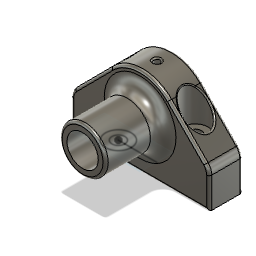
JKK60_WithCover_RailAdapter_12mm v9 (Autodesk Fusion 360 design; units mm, degrees)
Autodesk Fusion 360 part; units mm, degrees
note: some values were not read from the file. Chosen so that the rebuilt part matches the saved one: which face or edge a step refers to. Set by a fixed rule: which sketch regions a step uses.
sketch "Skizze1" plane through (0, 0, 0) normal (0, 0, 1) x (1, 0, 0)
  circle A0 centre (0, 0) radius 6
  line L0 (-27, -18.5) -> (0, -18.5)
  circle A1 centre (0, 0) radius 16
  line L1 (-27, -18.5) -> (-27, -4.5)
  line L2 (-27, -4.5) -> (-11.3594, 11.2678)
  line L3 (0, -18.5) -> (0, 0)
  circle A2 centre (0, 0) radius 16.5 construction
  line L4 (0, -16.5) -> (21.529, -16.5)
  line L5 (0, 0) -> (0, 20)
  circle A3 centre (62.865, -3.5125) radius 6
  circle A4 centre (62.865, -3.5125) radius 12.5
  line L6 (62.865, -3.5125) -> (62.865, -24.0125)
  line L7 (62.365, -24.0125) -> (92.365, -24.0125)
  circle A5 centre (62.865, -3.5125) radius 16.5 construction
  line L8 (62.865, -20.0125) -> (75, -20.0125) construction
  line L9 (50.365, -24.0125) -> (62.365, -24.0125)
  line L10 (92.365, -24.0125) -> (104.365, -24.0125)
  line L11 (68.6713, 7.5571) -> (104.365, -11.1649)
  line L12 (104.365, -11.1649) -> (104.365, -24.0125)
  line L13 (50.365, -3.5125) -> (50.365, -24.0125)
  point P0 (-15, -18.5)
  dimension "d1" = 12
  dimension "d3" = 32
  dimension "d4" = 33
  dimension "d5" = 2
  dimension "d6" = 27
  dimension "d7" = 15
  dimension "d8" = 12
  dimension "d9" = 25
  dimension "d10" = 30
  dimension "d11" = 33
  dimension "d12" = 4
  dimension "d13" = 54
  dimension "d14" = 12.8476
  dimension "d25" = 14
  constraint coincident A0.centre A1.centre
  constraint horizontal L0
  constraint concentric A0 A1
  constraint perpendicular L0 L1
  constraint vertical L3
  constraint concentric A0 A2
  constraint coincident L3 L4.start
  constraint perpendicular L3 L4
  constraint tangent A2 L4
  constraint coincident A1 L2.end
  constraint tangent A1 L2
  constraint coincident L0 P0
  constraint parallel L3 L5
  constraint concentric A3 A4
  constraint coincident A3.centre A4.centre
  constraint vertical L6
  constraint horizontal L7
  constraint coincident L6.end L7
  constraint concentric A4 A5
  constraint coincident L6 L8.start
  constraint perpendicular L6 L8
  constraint tangent A5 L8
  constraint perpendicular L6 L9
  constraint coincident L7.start L9.end
  constraint parallel L7 L10
  constraint equal L9 L10
  constraint coincident A4 L11.start
  constraint perpendicular L10 L12
  constraint tangent A4 L11
  constraint coincident A4 L13.start
  constraint vertical L13
  constraint tangent A4 L13
  measures "d1" diameter of A0
  measures "d3" diameter of A1
  measures "d4" diameter of A2
  measures "d5" distance of L0 L4
  measures "d6" distance of L0.start L0.end
  measures "d7" distance of L0.end P0
  measures "d8" diameter of A3
  measures "d9" diameter of A4
  measures "d10" distance of L7.start L7.end
  measures "d11" diameter of A5
  measures "d12" distance of L7 L8
  measures "d13" distance of L9.start L10.end
  measures "d14" distance of L10.end L11.end
  measures "d25" distance of L0.start L1.end
extrude "Extrusion1" add sketch "Skizze1" along normal blind 13 contours A0 A1 L3 L5 | L0 A1 L1 L2 L3 picked at (-9.646, 8.1637)
sketch "Skizze2" plane through (0, -18.5, 0) normal (0, -1, 0) x (1, 0, 0)
  line L0 (-27, 0) -> (0, 0)
  line L1 (0, 0) -> (0, 13)
  line L2 (0, 13) -> (-27, 13)
  line L3 (-27, 13) -> (-27, 0)
  line L4 (0, 6.5) -> (-15, 6.5)
  circle A0 centre (-15, 6.5) radius 2.5
  circle A1 centre (-15, 6.5) radius 5
  dimension "d17" = 5
  dimension "d18" = 10
  dimension "d37" = 15
  constraint midpoint L1 L4.start
  constraint perpendicular L1 L4
  constraint coincident L4.end A0.centre
  constraint concentric A0 A1
  measures "d17" diameter of A0
  measures "d18" diameter of A1
  measures "d37" distance of L4.start L4.end
extrude "Extrusion2" cut sketch "Skizze2" against normal blind 27 contours A0
ref_plane "Arbeitsebene1" through (-13.5, -1.5, 6.5) normal (0, -1, 0) x (1, 0, 0)
extrude "Extrusion3" cut sketch "Skizze2" against normal blind 27 from surface at -17 contours A0 | A1
mirror "Spiegeln1" about plane through (0, -16, 0) normal (1, 0, 0) of bodies 1 merged
sketch "Skizze3" plane through (11.3594, 11.2678, 0) normal (0.709965, 0.704237, 0) x (0, 0, -1)
  line L0 (0, -22.2092) -> (0, 0)
  line L1 (-9.9273, 0) -> (-13, 0)
  line L2 (-13, 0) -> (-13, -22.2092)
  line L3 (-13, -22.2092) -> (0, -22.2092)
  line L4 (0, -6) -> (0, 6)
  line L5 (0, 0) -> (-6.5, 0)
  circle A0 centre (-6.5, 0) radius 1.25
  line L6 (-6.5, 0) -> (-6.5, 5.407)
  ellipse E0 centre (-6.5, -5.1695) end of major axis (-6.5, 1.9304) minor radius 5 (-9.9273, 0) -> (-3.0727, 0) ccw
  line L7 (0, 0) -> (-3.0727, 0)
  dimension "d28" = 2.5
  constraint coincident L4 L0.end
  constraint perpendicular L4 L5
  constraint symmetric L4.start L4.end L5
  constraint coincident L5.end A0.centre
  constraint perpendicular L1 L6
  constraint symmetric L1.end L0.end L6
  measures "d28" diameter of A0
sketch "Skizze5" plane through (0, 0, 13) normal (0, 0, 1) x (1, 0, 0)
  arc A0 (11.3594, 11.2678) -> (-11.3594, 11.2678) centre (0, 0) ccw
  line L0 (-11.3594, 11.2678) -> (-27, -4.5)
  line L1 (-27, -4.5) -> (-27, -18.5)
  line L2 (-27, -18.5) -> (27, -18.5)
  line L3 (27, -18.5) -> (27, -4.5)
  line L4 (27, -4.5) -> (11.3594, 11.2678)
  circle A1 centre (0, 0) radius 6
  circle A2 centre (0, 0) radius 9
  dimension "d46" = 18
  constraint coincident A0.centre A1.centre
  measures "d46" diameter of A2
ref_plane "Arbeitsebene3" through (0, -1.25, 6.5) normal (0, 0, -1) x (-1, 0, 0)
ref_plane "Arbeitsebene4" through (0, -1.25, 35.5) normal (0, 0, -1) x (-1, 0, 0)
extrude "Extrusion6" add sketch "Skizze5" along normal up to surface (22.5 mm away) contours A2
fillet "Abrundung1" radius 5 2 edges at (-27, -4.5, 6.5) (27, -4.5, 6.5)
fillet "Abrundung6" radius 5 1 edges at (-8.3909, 3.2545, 13)
sketch "Skizze6" plane through (0, 0, 35.5) normal (0, 0, 1) x (1, 0, 0)
  circle A0 centre (0, 0) radius 6
  circle A1 centre (0, 0) radius 9
  circle A2 centre (0, 0) radius 6.1
  dimension "d52" = 0.1
extrude "Extrusion7" cut sketch "Skizze6" against normal up to surface (22.5 mm away) contours A0 | A2
fillet "Abrundung2" radius 1 19 edges at (27, -12.5296, 13) (0, -18.5, 13) (-27, -12.5296, 13) (-26.6233, -4.6552, 13) (-18.4546, 4.1149, 13) (0, 16, 13) (18.4546, 4.1149, 13) (26.6233, -4.6552, 13) (27, -12.5296, 0) (0, -18.5, 0) (-27, -12.5296, 0) (-26.6233, -4.6552, 0) (-18.4546, 4.1149, 0) (0, 16, 0) (18.4546, 4.1149, 0) (26.6233, -4.6552, 0) (-9, 0, 35.5) (6, 0, 0) (-6, 0, 0)
fillet "Abrundung5" radius 0.5 4 edges at (-10, 12.49, 6.5) (-20, 2.5569, 6.5) (10, 12.49, 6.5) (20, 2.5569, 6.5)
ref_plane "Arbeitsebene2" through (0, 21.5, 6.5) normal (0, -1, 0) x (1, 0, 0)
sketch "Skizze4" plane through (0, 21.5, 0) normal (0, -1, 0) x (-1, 0, 0)
  circle A0 centre (0, -6.5) radius 1.25
  point P0 (0, -6.5)
  dimension "d39" = 2.5
  constraint coincident P0 A0.centre
  measures "d39" diameter of A0
extrude "Extrusion5" cut sketch "Skizze4" along normal blind 19
fillet "Abrundung4" radius 0.5 1 edges at (-1.25, 15.9511, 6.5)
equation "d3 = d1 + 20 mm"
equation "d6 = ( 54 / 2 ) * 1 mm"
equation "d7 = ( 30 / 2 ) * 1 mm"
equation "d37 = ( 30 / 2 ) * 1 mm"
equation "d47 = -( ( 74 / 2 ) * 1 mm - 8 mm )"
